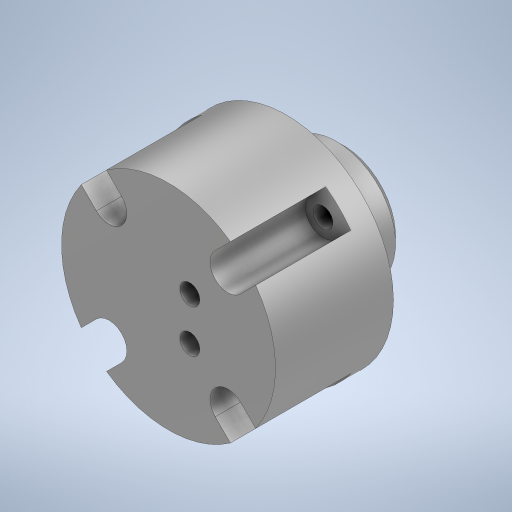
# Autodesk Inventor part: StageConnection
Saved by Autodesk Inventor 2023 (Build 270158000, 158)
## iProperties
Created: 2021-10-06
Part Number: StageConnection
Material: Aluminum 6061
Document SubType Name: Modeling
Designer: Timo
Density: 2.7 g/cm^3
Appearance: Anodized - Light Gray
Author: Timo
Autodesk Inventor part; units mm, degrees
ref_plane "YZ Plane" through (0, 0, 0) normal (1, 0, 0) x (0, 1, 0)
ref_plane "XZ Plane" through (0, 0, 0) normal (0, 1, 0) x (-1, 0, 0)
ref_plane "XY Plane" through (0, 0, 0) normal (0, 0, 1) x (1, 0, 0)
sketch "Sketch1" plane through (0, 0, 0) normal (0, 0, 1) x (1, 0, 0)
  circle A0 centre (0, 0) radius 22.5
  dimension "d0" = 45
  constraints: 1 centre point, 1 coincident
  measures "d0" diameter of A0
extrude "Extrusion1" add sketch "Sketch1" along normal blind 24.8
sketch "Sketch2" plane through (0, 0, 0) normal (0, 0, -1) x (-1, 0, 0)
  circle A0 centre (0, 0) radius 12.45
  dimension "d3" = 24.9
  constraints: 1 centre point, 1 coincident
  measures "d3" diameter of A0
extrude "Extrusion2" add sketch "Sketch2" along normal blind 12
sketch "Sketch3" plane through (0, 0, 24.8) normal (0, 0, 1) x (1, 0, 0)
  line L0 (12.5, -12.5) -> (-12.5, -12.5) construction
  line L1 (-12.5, -12.5) -> (-12.5, 12.5) construction
  line L2 (-12.5, 12.5) -> (12.5, 12.5) construction
  line L3 (12.5, 12.5) -> (12.5, -12.5) construction
  line L4 (12.5, -12.5) -> (-12.5, 12.5) construction
  line L5 (-12.5, -12.5) -> (12.5, 12.5) construction
  point P0 (0, 0)
  dimension "d6" = 25
  dimension "d7" = 25
  constraints: 12 end point, 2 midpoint, 2 parallel, 1 horizontal, 1 perpendicular
  measures "d6" distance of L1.end L2.end
  measures "d7" distance of L0.end L1.end
hole "Hole1" at (-12.5, 12.5, 24.8) at (12.5, 12.5, 24.8) at (12.5, -12.5, 24.8) at (-12.5, -12.5, 24.8) direction (0, 0, -1) diameter 4.2 end through all counterbore diameter 7.5 counterbore depth 20
sketch "Sketch4" plane through (0, 0, 24.8) normal (0, 0, 1) x (1, 0, 0)
  line L0 (-13.2583, 18.5616) -> (-9.8483, 15.1517)
  line L1 (-9.8483, 15.1517) -> (-15.1517, 9.8483)
  line L2 (-15.1517, 9.8483) -> (-18.5616, 13.2583)
  line L3 (-18.5616, 13.2583) -> (-13.2583, 18.5616)
  line L4 (-13.2583, 18.5616) -> (-15.1517, 9.8483) construction
  line L5 (-9.8483, 15.1517) -> (-18.5616, 13.2583) construction
  circle A0 centre (-12.5, 12.5) radius 3.75 projected
  circle A1 centre (0, 0) radius 22.5 projected
  circle A2 centre (-12.5, 12.5) radius 3.75 construction
  line L6 (-14.205, 14.205) -> (-12.5, 12.5) construction
  point P0 (-18.339, 13.0357)
  point P1 (-13.0357, 18.339)
  constraints: 14 end point, 3 midpoint, 2 parallel, 2 tangent, 1 coincident, 1 perpendicular, 1 point on line
extrude "Extrusion3" cut sketch "Sketch4" against normal up to surface (20 mm away) contours L0 A0 L2 A1 | L1 A0 picked at (-13.4167, 17.3703) picked at (-13.3264, 14.7238)
pattern_circular "Circular Pattern1" count 4 over 360 about axis through (0, 0, 0) along (0, 0, 1) of "Extrusion3"
chamfer "Chamfer1" distance 1.5 angle 45 1 edges at (12.45, 0, -12)
sketch "Sketch5" plane through (0, 0, -12) normal (0, 0, -1) x (-1, 0, 0)
  line L0 (0, 12) -> (-12, 12) construction
  line L1 (-12, 12) -> (-12, -32.1468) construction
  line L2 (-12, -32.1468) -> (0, -32.1468) construction
  line L3 (0, -32.1468) -> (0, 12) construction
  circle A0 centre (-4.5, 4.5) radius 3.75 construction
  circle A1 centre (-4.5, -4.5) radius 3.75 construction
  line L4 (-4.5, -4.5) -> (-4.5, 4.5) construction
  circle A2 centre (0, 0) radius 10.95 construction
  line L5 (31.5, 0) -> (-31.5, 0) construction
  dimension "d23" = 12
  dimension "d24" = 12
  dimension "d25" = 7.5
  dimension "d29" = 9
  dimension "d30" = 4.5
  constraints: 10 end point, 2 centre point, 2 coincident, 2 parallel, 1 equal radius, 1 horizontal, 1 perpendicular, 1 point on line, 1 vertical, 1 other
  measures "d23" distance of L0.start L0.end
  measures "d24" distance from line of point (0, 0) L0
  measures "d25" diameter of A0
  measures "d29" distance of L4.start L4.end
  measures "d30" distance from line of L3 L4.end
hole "Hole2" at (4.5, -4.5, -12) at (4.5, 4.5, -12) direction (0, 0, 1) diameter 4.2 end through all counterbore diameter 7.5 counterbore depth 30
body "Solid1"
